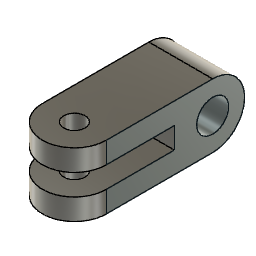
cad1 project (Autodesk Fusion 360 design; units mm, degrees)
Autodesk Fusion 360 part; units mm, degrees
sketch "Sketch1" plane through (0, 0, 0) normal (1, 0, 0) x (0, 1, 0)
  circle A0 centre (0, 0) radius 0.375
  arc A1 (0, -0.75) -> (0, 0.75) centre (0, 0) ccw
  line L0 (0, 0.75) -> (-2.4997, 0.75)
  line L1 (0, -0.75) -> (-2.5, -0.75)
  line L2 (-2.4997, 0.75) -> (-2.4997, 0.25)
  line L3 (-2.5, -0.75) -> (-2.5, -0.25)
  line L4 (-2.4997, 0.25) -> (-0.8997, 0.25)
  line L5 (-2.5, -0.25) -> (-0.9, -0.25)
  line L6 (-0.9, -0.25) -> (-0.8997, 0.25)
  dimension "d9" = 0.5
  dimension "d10" = 0.5
  dimension "d11" = 1.6
  dimension "d12" = 1.6
  constraint coincident A0.centre A1.centre
  constraint tangent A1 L0
  constraint horizontal L0
  constraint horizontal L1
  constraint perpendicular L0 L2
  constraint perpendicular L1 L3
  constraint perpendicular L2 L4
  constraint perpendicular L3 L5
  measures "d9" distance of L0.end L2.end
  measures "d10" distance of L1.end L3.end
  measures "d11" distance of L2.end L4.end
  measures "d12" distance of L3.end L5.end
extrude "Extrude1" add sketch "Sketch1" along normal blind 1.5
sketch "Sketch2" plane through (0, 0, 0.75) normal (0, 0, 1) x (-1, 0, 0)
  line L0 (0, 0) -> (0, 2.4997)
  line L1 (0, 2.4997) -> (-1.5, 2.4997)
  line L2 (-1.5, 2.4997) -> (-1.5, 0)
  line L3 (-1.5, 0) -> (0, 0)
  arc A0 (0, 2.4997) -> (-1.5, 2.4997) centre (-0.75, 2.4997) ccw
  line L4 (0, 2.4997) -> (-1.5, 2.4997)
  circle A1 centre (-0.75, 2.4997) radius 0.25
  dimension "d15" = 0.5
  constraint coincident L1.end L2.start
  constraint coincident L0.end L1.start
  constraint tangent L0 A0
  constraint concentric A0 A1
  measures "d15" diameter of A1
extrude "Extrude2" add sketch "Sketch2" against normal blind 0.5 contours L1 A0 L4 A1 | L1 L4 A1 picked at (-0.6889, 2.5564)
sketch "Sketch3" plane through (0, 0, 0.75) normal (0, 0, 1) x (-1, 0, 0)
  line L0 (0, 0) -> (0, 2.4997)
  arc A0 (0, 2.4997) -> (-1.5, 2.4997) centre (-0.75, 2.4997) ccw
  line L1 (-1.5, 2.4997) -> (-1.5, 0)
  line L2 (-1.5, 0) -> (0, 0)
  circle A1 centre (-0.75, 2.4997) radius 0.25
  dimension "d18" = 0.5
  constraint concentric A0 A1
  measures "d18" diameter of A1
extrude "Extrude3" cut sketch "Sketch3" against normal through all contours A1
sketch "Sketch4" plane through (0, 0, -0.75) normal (0, 0, -1) x (1, 0, 0)
  arc A0 (0.5, 2.5) -> (1, 2.5) centre (0.75, 2.4997) ccw
  line L0 (0.5, 2.5) -> (0, 2.5)
  line L1 (0, 2.5) -> (0, 0)
  line L2 (0, 0) -> (1.5, 0)
  line L3 (1.5, 0) -> (1.5, 2.5)
  line L4 (1.5, 2.5) -> (1, 2.5)
  line L5 (0, 2.5) -> (1.5, 2.5)
  arc A1 (1.5, 2.5) -> (0, 2.5) centre (0.75, 2.5) ccw
  circle A2 centre (0.75, 2.4997) radius 0.25
  dimension "d20" = 0.5
  constraint coincident L0.end L1.start
  constraint coincident L3.end L4.start
  constraint tangent L1 A1
  constraint concentric A0 A2
  measures "d20" diameter of A2
extrude "Extrude4" add sketch "Sketch4" against normal blind 0.5 contours L0 L4 L5 A1 A2
sketch "Sketch5" plane through (1.5, 0, 0) normal (1, 0, 0) x (0, 1, 0)
  circle A0 centre (0, 0) radius 0.375
  arc A1 (0, -0.75) -> (0, 0.75) centre (0, 0) ccw
  line L0 (0, 0.75) -> (-2.4997, 0.75)
  line L1 (-2.4997, 0.75) -> (-2.4997, 0.25)
  line L2 (-2.4997, 0.25) -> (-0.8997, 0.25)
  line L3 (-0.8997, 0.25) -> (-0.9, -0.25)
  line L4 (-0.9, -0.25) -> (-2.5, -0.25)
  line L5 (-2.5, -0.25) -> (-2.5, -0.75)
  line L6 (-2.5, -0.75) -> (0, -0.75)
  dimension "d23" = 2.4997
  dimension "d24" = 1.6
  dimension "d25" = 0.75
  measures "d23" distance of A1.end L0.end
  measures "d24" distance of L1.end L2.end
  measures "d25" diameter of A0
